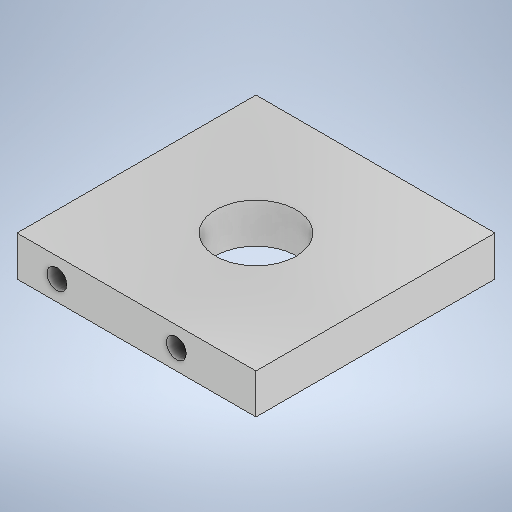
# Autodesk Inventor part: hand2_08
Saved by Autodesk Inventor 2025.1 (Build 291241000, 241)
## iProperties
Created: 2025-02-02
Part Number: hand2_08
Material: アルミニウム 6061-AHC
Document SubType Name: Modeling
Designer: ryogo
Density: 2.7 g/cm^3
Appearance: アルミニウム - ダーク
Author: ryogo
Autodesk Inventor part; units mm, degrees
ref_plane "YZ Plane" through (0, 0, 0) normal (1, 0, 0) x (0, 1, 0)
ref_plane "XZ Plane" through (0, 0, 0) normal (0, 1, 0) x (-1, 0, 0)
ref_plane "XY Plane" through (0, 0, 0) normal (0, 0, 1) x (1, 0, 0)
sketch "スケッチ1" plane through (0, 0, 0) normal (0, 1, 0) x (-1, 0, 0)
  line L0 (0, 0) -> (30, 0)
  line L1 (30, 0) -> (30, -30)
  line L2 (30, -30) -> (0, -30)
  line L3 (0, -30) -> (0, 0)
  dimension "d0" = 30
  dimension "d1" = 30
  constraints: 8 end point, 2 parallel, 1 horizontal, 1 perpendicular
  measures "d0" distance of L1.end L2.end
  measures "d1" distance of L0.end L1.end
extrude "押し出し1" add sketch "スケッチ1" along normal blind 5
sketch "スケッチ2" plane through (-30, 0, 0) normal (0, 0, 1) x (1, 0, 0)
  line L0 (0, 0) -> (0, 5) projected
  line L1 (0, 2.5) -> (30, 2.5)
  line L2 (30, 0) -> (30, 5) projected
  point P0 (5, 2.5)
  point P1 (20, 2.5)
  dimension "d4" = 10
  dimension "d5" = 15
  constraints: 2 end point, 2 midpoint, 2 point on line
  measures "d4" distance from line of L2 point (20, 2.5)
  measures "d5" distance of point (5, 2.5) point (20, 2.5)
hole "穴1" at (-25, 2.5, 0) at (-10, 2.5, 0) direction (0, 0, -1) diameter 2.5 end through all
sketch "スケッチ3" plane through (0, 5, 0) normal (0, 1, 0) x (1, 0, 0)
  line L0 (-30, 30) -> (-30, 0) projected
  line L1 (-30, 15) -> (0, 15)
  line L2 (0, 0) -> (0, 30) projected
  line L3 (-30, 0) -> (0, 0) projected
  line L4 (-15, 0) -> (-15, 30)
  line L5 (0, 30) -> (-30, 30) projected
  circle A0 centre (-15, 15) radius 5.05
  dimension "d13" = 10.1
  constraints: 5 midpoint, 4 end point, 1 centre point
  measures "d13" diameter of A0
extrude "押し出し2" cut sketch "スケッチ3" against normal blind 5 contours A0 L4 L1 | L1 L4 A0 | A0 L1 L4 | L1 A0 L4
